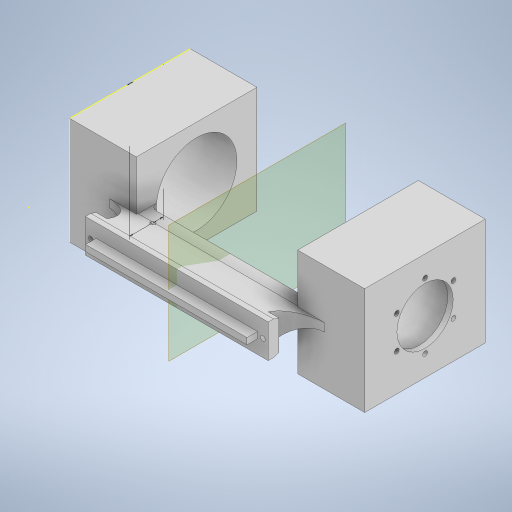
# Autodesk Inventor part: Bot v3 Wheel_Right
Saved by Autodesk Inventor 2024 (Build 280153000, 153)
## iProperties
Created: 2023-11-26
Part Number: Bot v3 Wheel_Right
Material: Generic
Document SubType Name: Modeling
Designer: CJ110
Density: 1 g/cm^3
Appearance: Default
Author: CJ110
Autodesk Inventor part; units mm, degrees
ref_plane "YZ Plane" through (0, 0, 0) normal (1, 0, 0) x (0, 1, 0)
ref_plane "XZ Plane" through (0, 0, 0) normal (0, 1, 0) x (-1, 0, 0)
ref_plane "XY Plane" through (0, 0, 0) normal (0, 0, 1) x (1, 0, 0)
sketch "Sketch1" plane through (0, 0, 0) normal (0, 1, 0) x (-1, 0, 0)
  line L0 (0, 0) -> (76.454, 0)
  line L1 (76.454, 0) -> (76.454, 25.4)
  line L2 (76.454, 25.4) -> (0, 25.4)
  line L3 (0, 25.4) -> (0, 0)
  dimension "d0" = 76.454
  dimension "d1" = 25.4
  constraints: 8 end point, 2 parallel, 1 horizontal, 1 perpendicular
  measures "d0" distance of L1.end L2.end
  measures "d1" distance between parallel lines of L0 L2
extrude "Extrusion1" add sketch "Sketch1" along normal blind 3.175
sketch "Sketch2" plane through (-76.454, 0, 25.4) normal (0, 0, 1) x (1, 0, 0)
  line L0 (-31.75, 26.9875) -> (0, 26.9875)
  line L1 (0, 26.9875) -> (0, -23.8125)
  line L2 (0, -23.8125) -> (-31.75, -23.8125)
  line L3 (-31.75, -23.8125) -> (-31.75, 26.9875)
  line L4 (76.454, 26.9875) -> (108.204, 26.9875)
  line L5 (108.204, 26.9875) -> (108.204, -23.8125)
  line L6 (108.204, -23.8125) -> (76.454, -23.8125)
  line L7 (76.454, -23.8125) -> (76.454, 26.9875)
  line L8 (0, 0) -> (0, 3.175) projected
  line L9 (-31.75, 1.5875) -> (108.204, 1.5875) construction
  line L10 (0, 0) -> (76.454, 0) projected
  line L11 (76.454, 0) -> (76.454, 3.175) projected
  line L12 (0, 3.175) -> (76.454, 3.175) projected
  line L13 (0, 0) -> (0, 3.175) projected
  point P0 (76.454, 0)
  point P1 (0, 1.5875)
  point P2 (0, 1.5875)
  dimension "d4" = 31.75
  dimension "d5" = 76.454
  dimension "d6" = 50.8
  dimension "d11" = 76.454
  constraints: 18 end point, 4 midpoint, 4 parallel, 3 horizontal, 2 collinear, 2 equal length, 2 perpendicular, 1 point on line
  measures "d4" distance between parallel lines of L1 L3
  measures "d5" distance between parallel lines of L7 L1
  measures "d6" distance between parallel lines of L2 L0
  measures "d11" distance of L12.start L11.end
extrude "Extrusion2" add sketch "Sketch2" along normal blind 50.8 contours L0 L1 L2 L3 | L7 L4 L5 L6
sketch "Sketch3" plane through (-76.454, 0, 25.4) normal (0, 0, -1) x (-1, 0, 0)
  line L0 (-76.454, 26.9875) -> (-76.454, 3.175) projected
  line L1 (-108.204, 26.9875) -> (-76.454, 26.9875) projected
  line L2 (-108.204, -23.8125) -> (-108.204, 26.9875) projected
  line L3 (-76.454, -23.8125) -> (-108.204, -23.8125) projected
  line L4 (-76.454, 0) -> (-76.454, -23.8125) projected
  line L5 (-76.454, 0) -> (-76.454, 3.175) projected
  line L6 (31.75, 26.9875) -> (31.75, -23.8125) projected
  line L7 (0, 26.9875) -> (31.75, 26.9875) projected
  line L8 (0, 3.175) -> (0, 26.9875) projected
  line L9 (0, 0) -> (0, 3.175) projected
  line L10 (0, -23.8125) -> (0, 0) projected
  line L11 (31.75, -23.8125) -> (0, -23.8125) projected
  point P0 (-76.454, 0)
extrude "Extrusion3" add sketch "Sketch3" along normal blind 6.35
fillet "Fillet3" radius 3.175 2 edges at (-76.454, 1.5875, 25.4) (0, 1.5875, 25.4)
sketch "Sketch4" plane through (31.75, -23.8125, 76.2) normal (1, 0, 0) x (0, 0, -1)
  circle A0 centre (28.575, 25.4) radius 13.335
  line L0 (57.15, 50.8) -> (0, 50.8) projected
  line L1 (28.575, 50.8) -> (28.575, 0) construction
  line L2 (0, 0) -> (57.15, 0) projected
  line L3 (0, 50.8) -> (0, 0) projected
  line L4 (0, 25.4) -> (57.15, 25.4) construction
  circle A1 centre (28.575, 40.894) radius 1.143
  circle A2 centre (15.1568, 33.147) radius 1.143
  circle A3 centre (15.1568, 17.653) radius 1.143
  circle A4 centre (28.575, 9.906) radius 1.143
  circle A5 centre (41.9932, 17.653) radius 1.143
  circle A6 centre (41.9932, 33.147) radius 1.143
  line L5 (57.15, 50.8) -> (0, 50.8) projected
  line L6 (0, 0) -> (0, 50.8) projected
  point P0 (76.2, 23.8125)
  dimension "d15" = 26.67
  dimension "d16" = 15.494
  dimension "d17" = 2.286
  dimension "d20" = 360
  constraints: 8 midpoint, 7 centre point, 4 end point, 1 horizontal, 1 point on line, 13 other
  measures "d15" diameter of A0
  measures "d16" distance of point (28.575, 25.4) A1.centre
  measures "d17" diameter of A1
extrude "Extrusion4" cut sketch "Sketch4" against normal through all
ref_plane "Work Plane1" through (-38.227, -23.8125, 76.2) normal (1, 0, 0) x (0, 0, -1)
sketch "Sketch5" plane through (-38.227, -23.8125, 76.2) normal (1, 0, 0) x (0, 0, -1)
  circle A0 centre (28.575, 25.4) radius 13.335 projected
  circle A1 centre (28.575, 25.4) radius 19.05
  point P0 (76.2, 23.8125)
  dimension "d24" = 38.1
  constraints: 1 centre point, 1 coincident
  measures "d24" diameter of A1
extrude "Extrusion5" cut sketch "Sketch5" along normal mid plane 134.874 contours A0 | A1
sketch "Sketch7" plane through (-38.227, -23.8125, 76.2) normal (1, 0, 0) x (0, 0, -1)
  line L0 (73.66, 33.3375) -> (56.2135, 26.9875)
  line L1 (73.66, 17.4625) -> (56.2135, 23.8125)
  line L2 (76.2, 23.8125) -> (76.2, 26.9875) projected
  line L3 (76.2, 26.8875) -> (81.18, 26.8875)
  line L4 (81.18, 26.8875) -> (81.18, 23.9125)
  line L5 (81.18, 23.9125) -> (76.2, 23.9125)
  line L6 (76.2, 23.8125) -> (57.15, 23.8125) projected
  line L7 (57.15, 23.8125) -> (76.2, 23.8125) projected
  line L8 (47.625, 23.8125) -> (57.15, 23.8125) projected
  line L9 (50.8, 23.8125) -> (47.625, 23.8125) projected
  line L10 (47.625, 23.8125) -> (50.8, 23.8125) projected
  line L11 (57.15, 23.8125) -> (47.625, 23.8125) projected
  line L12 (76.2, 26.9875) -> (57.15, 26.9875) projected
  line L13 (57.15, 26.9875) -> (47.625, 26.9875) projected
  line L14 (50.8, 26.9875) -> (47.625, 26.9875) projected
  line L15 (47.625, 26.9875) -> (50.8, 26.9875) projected
  line L16 (47.625, 26.9875) -> (57.15, 26.9875) projected
  line L17 (57.15, 26.9875) -> (76.2, 26.9875) projected
  line L18 (73.66, 33.3375) -> (73.66, 26.9875)
  line L19 (73.66, 33.3375) -> (76.2, 33.3375)
  line L20 (76.2, 33.3375) -> (76.2, 26.9875)
  line L21 (73.66, 17.4625) -> (73.66, 23.8125)
  line L22 (73.66, 17.4625) -> (76.2, 17.4625)
  line L23 (76.2, 17.4625) -> (76.2, 23.8125)
  point P0 (59.8682, 23.8125)
  point P1 (58.7535, 26.9875)
  dimension "d38" = 4.98
  dimension "d48" = 0.1
  dimension "d49" = 0.1
  dimension "d58" = 2.54
  dimension "d60" = 6.35
  dimension "d61" = 70
  dimension "d62" = 70
  constraints: 22 end point, 6 perpendicular, 6 point on line, 2 equal length, 2 horizontal, 1 vertical
  measures "d38" distance between parallel lines of L2 L4
  measures "d48" distance between parallel lines of L17 L3
  measures "d49" distance between parallel lines of L7 L5
  measures "d58" distance of L0.start L19.end
  measures "d60" distance between parallel lines of L17 L19
  measures "d61" angle of L0 L18
  measures "d62" angle of L21 L1
extrude "Extrusion8" add sketch "Sketch7" along normal mid plane 76.454
sketch "Sketch10" plane through (0, 0, 19.05) normal (1, 0, 0) x (0, 0, -1)
  line L0 (0, -0.3409) -> (0, 3.5159) projected
  line L1 (19.05, -6.35) -> (19.05, 0.1) projected
  line L2 (19.05, 0.1) -> (24.03, 0.1) projected
  line L3 (24.03, 0.1) -> (24.03, 3.075) projected
  line L4 (24.03, 3.075) -> (19.05, 3.075) projected
  line L5 (19.05, 3.075) -> (19.05, 9.525) projected
  line L6 (16.51, 9.525) -> (0, 3.5159) projected
  line L7 (0, 3.5159) -> (16.51, 9.525) projected
  line L8 (13.97, 8.6005) -> (13.97, -5.4255)
  line L9 (16.51, -6.35) -> (0, -0.3409) projected
  line L10 (19.05, 3.075) -> (19.05, 0.1)
  line L11 (19.05, 9.525) -> (16.51, 9.525) projected
  line L12 (0, -0.3409) -> (16.51, -6.35) projected
  line L13 (16.51, -6.35) -> (19.05, -6.35) projected
  point P0 (19.05, 0)
  point P1 (13.97, 8.6005)
  point P2 (13.97, 8.443)
  dimension "d50" = 5.08
  constraints: 4 end point, 2 point on line, 1 vertical
  measures "d50" distance between parallel lines of L5 L8
extrude "Extrusion9" add sketch "Sketch10" along normal blind 5.08 contours L8 L6 L11 L5 L10 L1 L13 L9
sketch "Sketch11" plane through (0, 3.075, 0) normal (0, 0, -1) x (-1, 0, 0)
  circle A0 centre (-2.54, -1.4875) radius 1.143
  line L0 (-5.08, 5.5255) -> (-5.08, -8.5005) projected
  line L1 (-5.08, -1.4875) -> (0, -1.4875) construction
  line L2 (0, 0) -> (76.454, 0) projected
  line L3 (0, -2.975) -> (0, 0) projected
  line L4 (76.454, -2.975) -> (0, -2.975) projected
  line L5 (76.454, 0) -> (76.454, -2.975) projected
  point P0 (0, -3.075)
  point P1 (-5.08, -7.576)
  dimension "d53" = 2.286
  dimension "d54" = 2.54
  constraints: 3 midpoint, 2 end point, 1 centre point, 1 horizontal
  measures "d53" diameter of A0
  measures "d54" distance from line of L0 A0.centre
extrude "Extrusion10" cut sketch "Sketch11" against normal up to surface (5.08 mm away) contours A0
mirror "Mirror1" about plane through (-38.227, -23.8125, 76.2) normal (1, 0, 0) of "Extrusion10", "Extrusion9"
fillet "Fillet4" radius 12.7 2 edges at (0, 1.5875, 19.05) (-76.454, 1.5875, 19.05)
sketch "Sketch12" plane through (31.75, -23.8125, 76.2) normal (1, 0, 0) x (0, 0, -1)
  circle A0 centre (15.1568, 17.653) radius 1.143 projected
  circle A1 centre (28.575, 25.4) radius 13.335 projected
  circle A2 centre (41.9932, 33.147) radius 1.143 projected
  circle A3 centre (15.1568, 33.147) radius 1.143 projected
  circle A4 centre (28.575, 9.906) radius 1.143 projected
  circle A5 centre (41.9932, 17.653) radius 1.143 projected
  circle A6 centre (28.575, 40.894) radius 1.143 projected
  line L0 (57.15, 50.8) -> (0, 50.8) projected
  line L1 (0, 0) -> (0, 50.8) projected
  line L2 (57.15, 0) -> (0, 0) projected
  line L3 (57.15, 50.8) -> (57.15, 0) projected
  circle A7 centre (28.575, 25.4) radius 25.4
  line L4 (12.7, 50.8) -> (12.7, 0)
  point P0 (76.2, 23.8125)
  dimension "d63" = 15.875
  constraints: 2 end point, 2 point on line, 1 centre point, 1 coincident, 1 tangent, 1 vertical
  measures "d63" distance from line of L4 A1.centre
equation "\"d5\" = d11"
equation "\"d62\" = d61"
body "Solid1"
